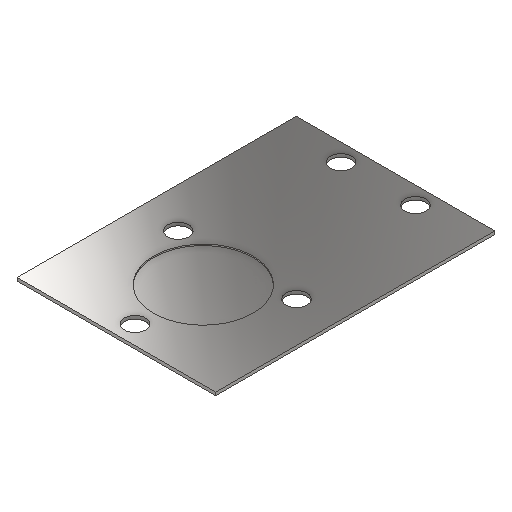
# Autodesk Inventor part: B_holder_sub_5
Saved by Autodesk Inventor 2026.2 (Build 302298000, 298)
## iProperties
Created: 2026-02-20
Part Number: B_holder_sub_5
Material: ステンレス鋼 440C
Document SubType Name: Modeling
Designer: zetsu
Density: 7.75 g/cm^3
Appearance: 半つや出し
Author: zetsu
Autodesk Inventor part; units mm, degrees
ref_plane "YZ Plane" through (0, 0, 0) normal (1, 0, 0) x (0, 1, 0)
ref_plane "XZ Plane" through (0, 0, 0) normal (0, 1, 0) x (-1, 0, 0)
ref_plane "XY Plane" through (0, 0, 0) normal (0, 0, 1) x (1, 0, 0)
sketch "スケッチ1" plane through (0, 0, 0) normal (0, 1, 0) x (-1, 0, 0)
  line L0 (16, -31) -> (16, 14)
  line L1 (16, 14) -> (-16, 14)
  line L2 (-16, 14) -> (-16, -31)
  line L3 (-16, -31) -> (16, -31)
  line L4 (0, 0) -> (0, -32.6995) construction
  point P0 (0, 14)
  dimension "d0" = 45
  dimension "d1" = 32
  dimension "d2" = 14
  constraints: 10 end point, 3 perpendicular, 2 vertical, 1 midpoint, 1 other
  measures "d0" distance of L0.end L0.start
  measures "d1" distance of L1.end L0.end
  measures "d2" distance of point (0, 14) L4.start
extrude "押し出し1" add sketch "スケッチ1" along normal blind 0.5
sketch "スケッチ4" plane through (0, 0.5, 0) normal (0, 1, 0) x (1, 0, 0)
  circle A0 centre (0, -11) radius 1.7
  line L0 (0, 0) -> (-18.7084, 0) construction
  circle A1 centre (-6, 28.2) radius 1.7
  circle A2 centre (6, 28.2) radius 1.7
  line L1 (0, 0) -> (0, 29.6633) construction
  line L2 (16, 31) -> (-16, 31) projected
  circle A3 centre (9.5263, 5.5) radius 1.7
  circle A4 centre (-9.5263, 5.5) radius 1.7
  point P0 (0, 31)
  dimension "d12" = 3.4
  dimension "d35" = 3.4
  dimension "d36" = 3.4
  dimension "d37" = 6
  dimension "d38" = 2.8
  dimension "d39" = 11
  dimension "d42" = 360
  constraints: 5 centre point, 4 end point, 1 horizontal, 1 midpoint, 1 symmetric about line, 1 vertical, 7 other
  measures "d12" diameter of A0
  measures "d35" diameter of A1
  measures "d36" diameter of A2
  measures "d37" horizontal distance of A2.centre L0.start
  measures "d38" vertical distance of point (0, 31) A2.centre
  measures "d39" distance of A0.centre L0.start
extrude "押し出し3" cut sketch "スケッチ4" against normal through all
sketch "スケッチ6" plane through (0, 0.5, 0) normal (0, 1, 0) x (1, 0, 0)
  circle A0 centre (0, 0) radius 8
  dimension "d44" = 16
  constraints: 1 centre point, 1 coincident
  measures "d44" diameter of A0
extrude "押し出し5" cut sketch "スケッチ6" against normal blind 0.2
